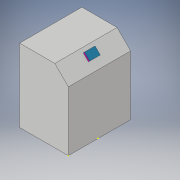
# Autodesk Inventor part: Ventilator
Saved by Autodesk Inventor 2019 (Build 230136000, 136)
## iProperties
Created: 2020-04-09
Part Number: Ventilator
Material: Generic
Document SubType Name: Modeling
Designer: MO_WIZZ
Density: 1 g/cm^3
Appearance: Default
Author: MO_WIZZ
Autodesk Inventor part; units mm, degrees
ref_plane "YZ Plane" through (0, 0, 0) normal (1, 0, 0) x (0, 1, 0)
ref_plane "XZ Plane" through (0, 0, 0) normal (0, 1, 0) x (-1, 0, 0)
ref_plane "XY Plane" through (0, 0, 0) normal (0, 0, 1) x (1, 0, 0)
sketch "Sketch1" plane through (0, 0, 0) normal (0, 1, 0) x (-1, 0, 0)
  line L0 (0, 0) -> (36, 0)
  line L1 (36, 0) -> (36, -46)
  line L2 (36, -46) -> (0, -46)
  line L3 (0, -46) -> (0, 0)
  dimension "d0" = 46
  dimension "d1" = 36
  constraints: 8 end point, 2 parallel, 1 horizontal, 1 perpendicular
  measures "d0" distance of L0.end L1.end
  measures "d1" distance of L1.end L2.end
extrude "Extrusion1" add sketch "Sketch1" along normal blind 54
chamfer "Chamfer1" distance 10 angle 45 1 edges at (0, 54, -23)
sketch "Sketch2" plane through (-36, 0, 0) normal (0, 0, 1) x (1, 0, 0)
  point P0 (36, 0)
sketch "Sketch3" plane through (-10, 54, -46) normal (0.7071, 0.7071, 0) x (-0.7071, 0.7071, 0)
  line L0 (-2.5891, 26.7922) -> (-8.0891, 26.7922)
  line L1 (-8.0891, 26.7922) -> (-8.0891, 18.7922)
  line L2 (-8.0891, 18.7922) -> (-2.5891, 18.7922)
  line L3 (-2.5891, 18.7922) -> (-2.5891, 26.7922)
  line L4 (-19.799, 46) -> (18.3848, 46) projected
  point P0 (-45.2548, 46)
  dimension "d7" = 8
  dimension "d8" = 5.5
  constraints: 8 end point, 2 parallel, 1 horizontal, 1 perpendicular
  measures "d7" distance of L2.end L0.start
  measures "d8" distance of L1.end L2.end
extrude "Extrusion2" add sketch "Sketch3" along normal blind 1
sketch "Sketch4" plane through (-10, 54, -46) normal (0.7071, 0.7071, 0) x (-0.7071, 0.7071, 0)
  point P0 (-45.2548, 46)
sketch "Sketch5" plane through (-36, 0, 0) normal (0, 0, 1) x (1, 0, 0)
  point P0 (36, 0)
body "Solid1"
